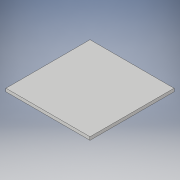
# Autodesk Inventor part: Tabs 1 inch
Saved by Autodesk Inventor 2017.3 (Build 213256000, 256)
## iProperties
Created: 2019-02-14
Part Number: Tabs 1 inch
Material: Generic
Document SubType Name: Modeling
Designer: LSabe
Density: 1 g/cm^3
Appearance: Default
Author: LSabe
Autodesk Inventor part; units mm, degrees
ref_plane "YZ Plane" through (0, 0, 0) normal (1, 0, 0) x (0, 1, 0)
ref_plane "XZ Plane" through (0, 0, 0) normal (0, 1, 0) x (-1, 0, 0)
ref_plane "XY Plane" through (0, 0, 0) normal (0, 0, 1) x (1, 0, 0)
sketch "Sketch1" plane through (0, 0, 0) normal (0, 0, 1) x (1, 0, 0)
  line L0 (82.55, 12.2094) -> (44.45, 12.2094)
  line L1 (44.45, 12.2094) -> (63.5, 12.2094)
  line L2 (82.55, 12.2094) -> (82.55, 10.8124)
  line L3 (82.55, 10.8124) -> (44.45, 10.8124)
  line L4 (44.45, 10.8124) -> (44.45, 12.2094)
  constraints: 10 end point, 2 horizontal, 2 parallel, 1 perpendicular
extrude "Extrusion1" add sketch "Sketch1" along normal blind 38.1
body "Solid1"
